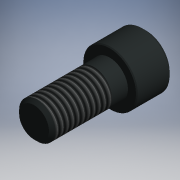
# Autodesk Inventor part: DIN-912 - M12x25(F)
Saved by Autodesk Inventor 2017.3 (Build 213256000, 256)
## iProperties
Part Number: DIN-912 - M12x25(F)
Material: Generic
Catalog Web Link: www.cadenas.de
Description: DIN-912-Cylinder screw
Vendor: FESTO
Document SubType Name: Modeling
Designer: partserver
Manufacturer: FESTO
Mass: 5.22026 g
Surface Area: 22.6144 cm^2
Volume: 5.22026 cm^3
Density: 1 g/cm^3
Appearance: PSOLRGB-45-51-51
Category: PARTsolutions
Company: FESTO
Title: DIN-912 - M12x25(F)
Author: Cadenas PARTsolutions
Comments: Cylinder screw
PSOL_IDENT_0: {$CADENAS_DATA\23d-libs\festo\zyl_zubeh\d912\din_912.prj},180 {VTYP=3D},{NB=DIN-912 - M12x25(F)},{LI
PSOL_IDENT_1: NA=DIN-912 - M12x25(F)},{NN=DIN-912},{DATE=01.07.2020 05:33:41},{GEOMDATE=01.07.2020 05:33:34},{VERS
PSOL_IDENT_2: ION=},{LINEID=870},{WBVAR=},{WBNUMERIC=}  {NB=DIN-912 - M12x25(F)},{LINA=DIN-912 - M12x25(F)},{KT=X}
PSOL_IDENT_3: ,{IDNR=},{GEW=M12},{DG=12.000},{P=1.750},{L=25.000},{B=25.000},{FORM=1},{GKD=9.853},{DK=18.000},{DAD
PSOL_IDENT_4: IN=13.700},{DS=12.000},{E=11.430},{LF=1.870},{K=12.000},{R=0.600},{S=10.000},{T=6.000},{V=1.200},{DW=
PSOL_IDENT_5: 17.230},{W=4.800},{NENN=M12x25},{DA=12.1},{BL=19.75}
NB: DIN-912 - M12x25(F)
NN: DIN-912
NT: Cylinder screw
NBSYN: DIN-912 - $NENN.(F)
LINA: DIN-912 - M12x25(F)
CATALOG: Festo
ROWDESC: M12x25
GEW: M12
DG: 12
P: 1.75
L: 25
B: 25
FORM: 1
GKD: 9.853
DK: 18
DADIN: 13.7
DS: 12
E: 11.43
LF: 1.87
K: 12
R: 0.6
S: 10
T: 6
V: 1.2
DW: 17.23
W: 4.8
SUPPLIER: FESTO
ARTICLENO: DIN-912 - M12x25(F)
BOMINFO: DIN-912 - M12x25(F)
CREATOR: CADENAS GmbH
Autodesk Inventor part; units mm, degrees
sketch "Sketch_1" plane through (0, 0, 0) normal (0, 0, 1) x (1, 0, 0)
  line L0 (0, -25) -> (0, 12)
  line L1 (0, 3.1132) -> (5, 6)
  line L2 (5, 6) -> (5, 11.2265)
  line L3 (5, 11.2265) -> (5.7735, 12)
  line L4 (5.7735, 12) -> (7.8, 12)
  line L5 (7.8, 12) -> (9, 10.8)
  line L6 (9, 10.8) -> (9, 0.3)
  line L7 (9, 0.3) -> (8.7, 0)
  line L8 (8.7, 0) -> (6.05, 0)
  line L9 (6.05, 0) -> (6, -1.87)
  line L10 (6, -1.87) -> (6, -23.9265)
  line L11 (6, -23.9265) -> (4.9265, -25)
  line L12 (4.9265, -25) -> (0, -25)
  line L13 (0, -25) -> (0, 3.1132)
  constraints: 28 end point
revolve "Revolution1" add sketch "Sketch_1" angle 360 about axis through (0, -25, 0) along (0, -1, 0)
thread "Thread1" size "M12x1.75" class "6g" standard "ISO Metric profile" length 18.6765
sketch "Sketch_2" plane through (0, 12, 0) normal (0, 1, 0) x (1, 0, 0)
  line L0 (-5, -2.8868) -> (0, -5.7735)
  line L1 (0, -5.7735) -> (5, -2.8868)
  line L2 (5, -2.8868) -> (5, 2.8868)
  line L3 (5, 2.8868) -> (0, 5.7735)
  line L4 (0, 5.7735) -> (-5, 2.8868)
  line L5 (-5, 2.8868) -> (-5, -2.8868)
  constraints: 12 end point
extrude "Extrusion1" cut sketch "Sketch_2" against normal blind 6
ref_plane "ANBAU_XY" through (0, 0, 0) normal (0, 1, 0) x (1, 0, 0)
ref_plane "ANBAU_YZ" through (0, 0, 0) normal (1, 0, 0) x (0, 0, -1)
ref_plane "ANBAU_ZX" through (0, 0, 0) normal (0, 0, -1) x (0, 1, 0)
ref_plane "Schraube_XY" through (0, 0, 0) normal (0, 1, 0) x (1, 0, 0)
ref_plane "Schraube_YZ" through (0, 0, 0) normal (1, 0, 0) x (0, 0, -1)
ref_plane "Schraube_ZX" through (0, 0, 0) normal (0, 0, -1) x (0, 1, 0)
ref_plane "insert_XY" through (0, 0, 0) normal (0, 1, 0) x (1, 0, 0)
ref_plane "insert_YZ" through (0, 0, 0) normal (1, 0, 0) x (0, 0, -1)
ref_plane "insert_ZX" through (0, 0, 0) normal (0, 0, -1) x (0, 1, 0)
ref_plane "schrauben_punkt_XY" through (0, -25, 0) normal (0, 1, 0) x (1, 0, 0)
ref_plane "schrauben_punkt_YZ" through (0, -25, 0) normal (1, 0, 0) x (0, 0, -1)
ref_plane "schrauben_punkt_ZX" through (0, -25, 0) normal (0, 0, -1) x (0, 1, 0)
body "Solid1"
